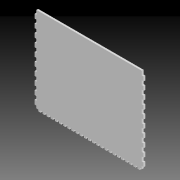
# Autodesk Inventor part: KB33-046-004-016 - Крышка
Saved by Autodesk Inventor 2020 (Build 240168000, 168)
## iProperties
Created: 2021-06-26
Part Number: KB33-046-004-016 - Крышка
Material: Типовые
Document SubType Name: Modeling
Designer: Петров Иван
Mass: 215.32 g
Surface Area: 1127.88 cm^2
Volume: 215.32 cm^3
Density: 1 g/cm^3
Appearance: По умолчанию
Author: Петров Иван
Autodesk Inventor part; units mm, degrees
ref_plane "YZ Plane" through (0, 0, 0) normal (1, 0, 0) x (0, 1, 0)
ref_plane "XZ Plane" through (0, 0, 0) normal (0, 1, 0) x (-1, 0, 0)
ref_plane "XY Plane" through (0, 0, 0) normal (0, 0, 1) x (1, 0, 0)
sketch "Эскиз1" plane through (0, 0, 0) normal (0, 0, 1) x (1, 0, 0)
  line L0 (0, 16.0005) -> (-4, 16.0005) projected
  line L1 (-4, 6.0005) -> (-4, 16.0005) projected
  line L2 (-4, 6.0005) -> (0, 6.0005) projected
  line L3 (0, 16.0005) -> (0, 6.0005) projected
  line L4 (0, 36.0005) -> (-4, 36.0005) projected
  line L5 (-4, 26.0005) -> (-4, 36.0005) projected
  line L6 (-4, 26.0005) -> (0, 26.0005) projected
  line L7 (0, 36.0005) -> (0, 26.0005) projected
  line L8 (0, 56.0005) -> (-4, 56.0005) projected
  line L9 (-4, 46.0005) -> (-4, 56.0005) projected
  line L10 (-4, 46.0005) -> (0, 46.0005) projected
  line L11 (0, 56.0005) -> (0, 46.0005) projected
  line L12 (0, 196.0005) -> (-4, 196.0005) projected
  line L13 (-4, 186.0005) -> (-4, 196.0005) projected
  line L14 (-4, 186.0005) -> (0, 186.0005) projected
  line L15 (0, 196.0005) -> (0, 186.0005) projected
  line L16 (0, 176.0005) -> (-4, 176.0005) projected
  line L17 (-4, 166.0005) -> (-4, 176.0005) projected
  line L18 (-4, 166.0005) -> (0, 166.0005) projected
  line L19 (0, 176.0005) -> (0, 166.0005) projected
  line L20 (0, 156.0005) -> (-4, 156.0005) projected
  line L21 (-4, 146.0005) -> (-4, 156.0005) projected
  line L22 (-4, 146.0005) -> (0, 146.0005) projected
  line L23 (0, 156.0005) -> (0, 146.0005) projected
  line L24 (0, 116.0005) -> (-4, 116.0005) projected
  line L25 (-4, 106.0005) -> (-4, 116.0005) projected
  line L26 (-4, 106.0005) -> (0, 106.0005) projected
  line L27 (0, 116.0005) -> (0, 106.0005) projected
  line L28 (0, 136.0005) -> (-4, 136.0005) projected
  line L29 (-4, 126.0005) -> (-4, 136.0005) projected
  line L30 (-4, 126.0005) -> (0, 126.0005) projected
  line L31 (0, 136.0005) -> (0, 126.0005) projected
  line L32 (0, 96.0005) -> (-4, 96.0005) projected
  line L33 (-4, 86.0005) -> (-4, 96.0005) projected
  line L34 (-4, 86.0005) -> (0, 86.0005) projected
  line L35 (0, 96.0005) -> (0, 86.0005) projected
  line L36 (0, 76.0005) -> (-4, 76.0005) projected
  line L37 (-4, 66.0005) -> (-4, 76.0005) projected
  line L38 (-4, 66.0005) -> (0, 66.0005) projected
  line L39 (0, 76.0005) -> (0, 66.0005) projected
  line L40 (-194, 0) -> (-194, -4) projected
  line L41 (-189, -4) -> (-194, -4) projected
  line L42 (-189, -4) -> (-189, 0) projected
  line L43 (-194, 0) -> (-189, 0) projected
  line L44 (-184, 0) -> (-184, -4) projected
  line L45 (-179, -4) -> (-184, -4) projected
  line L46 (-179, -4) -> (-179, 0) projected
  line L47 (-184, 0) -> (-179, 0) projected
  line L48 (-174, 0) -> (-174, -4) projected
  line L49 (-169, -4) -> (-174, -4) projected
  line L50 (-169, -4) -> (-169, 0) projected
  line L51 (-174, 0) -> (-169, 0) projected
  line L52 (-164, 0) -> (-164, -4) projected
  line L53 (-159, -4) -> (-164, -4) projected
  line L54 (-159, -4) -> (-159, 0) projected
  line L55 (-164, 0) -> (-159, 0) projected
  line L56 (-154, 0) -> (-154, -4) projected
  line L57 (-149, -4) -> (-154, -4) projected
  line L58 (-149, -4) -> (-149, 0) projected
  line L59 (-154, 0) -> (-149, 0) projected
  line L60 (-144, 0) -> (-144, -4) projected
  line L61 (-139, -4) -> (-144, -4) projected
  line L62 (-139, -4) -> (-139, 0) projected
  line L63 (-144, 0) -> (-139, 0) projected
  line L64 (-14, 0) -> (-14, -4) projected
  line L65 (-9, -4) -> (-14, -4) projected
  line L66 (-9, -4) -> (-9, 0) projected
  line L67 (-14, 0) -> (-9, 0) projected
  line L68 (-24, 0) -> (-24, -4) projected
  line L69 (-19, -4) -> (-24, -4) projected
  line L70 (-19, -4) -> (-19, 0) projected
  line L71 (-24, 0) -> (-19, 0) projected
  line L72 (-95.712, 271.7663) -> (-95.712, 277.9752) projected
  line L73 (-34, 0) -> (-34, -4) projected
  line L74 (-29, -4) -> (-34, -4) projected
  line L75 (-29, -4) -> (-29, 0) projected
  line L76 (-34, 0) -> (-29, 0) projected
  line L77 (-44, 0) -> (-44, -4) projected
  line L78 (-39, -4) -> (-44, -4) projected
  line L79 (-39, -4) -> (-39, 0) projected
  line L80 (-44, 0) -> (-39, 0) projected
  line L81 (-54, 0) -> (-54, -4) projected
  line L82 (-49, -4) -> (-54, -4) projected
  line L83 (-49, -4) -> (-49, 0) projected
  line L84 (-54, 0) -> (-49, 0) projected
  line L85 (-64, 0) -> (-64, -4) projected
  line L86 (-59, -4) -> (-64, -4) projected
  line L87 (-59, -4) -> (-59, 0) projected
  line L88 (-64, 0) -> (-59, 0) projected
  line L89 (-74, 0) -> (-74, -4) projected
  line L90 (-69, -4) -> (-74, -4) projected
  line L91 (-69, -4) -> (-69, 0) projected
  line L92 (-74, 0) -> (-69, 0) projected
  line L93 (-84, 0) -> (-84, -4) projected
  line L94 (-79, -4) -> (-84, -4) projected
  line L95 (-79, -4) -> (-79, 0) projected
  line L96 (-84, 0) -> (-79, 0) projected
  line L97 (-94, 0) -> (-94, -4) projected
  line L98 (-89, -4) -> (-94, -4) projected
  line L99 (-89, -4) -> (-89, 0) projected
  line L100 (-94, 0) -> (-89, 0) projected
  line L101 (-104, 0) -> (-104, -4) projected
  line L102 (-99, -4) -> (-104, -4) projected
  line L103 (-99, -4) -> (-99, 0) projected
  line L104 (-104, 0) -> (-99, 0) projected
  line L105 (-114, 0) -> (-114, -4) projected
  line L106 (-109, -4) -> (-114, -4) projected
  line L107 (-109, -4) -> (-109, 0) projected
  line L108 (-114, 0) -> (-109, 0) projected
  line L109 (-134, 0) -> (-134, -4) projected
  line L110 (-129, -4) -> (-134, -4) projected
  line L111 (-129, -4) -> (-129, 0) projected
  line L112 (-134, 0) -> (-129, 0) projected
  line L113 (-124, 0) -> (-124, -4) projected
  line L114 (-119, -4) -> (-124, -4) projected
  line L115 (-119, -4) -> (-119, 0) projected
  line L116 (-124, 0) -> (-119, 0) projected
  line L117 (-259, 16.0005) -> (-263, 16.0005) projected
  line L118 (-263, 6.0005) -> (-263, 16.0005) projected
  line L119 (-263, 6.0005) -> (-259, 6.0005) projected
  line L120 (-259, 16.0005) -> (-259, 6.0005) projected
  line L121 (-259, 36.0005) -> (-263, 36.0005) projected
  line L122 (-263, 26.0005) -> (-263, 36.0005) projected
  line L123 (-263, 26.0005) -> (-259, 26.0005) projected
  line L124 (-259, 36.0005) -> (-259, 26.0005) projected
  line L125 (-259, 56.0005) -> (-263, 56.0005) projected
  line L126 (-263, 46.0005) -> (-263, 56.0005) projected
  line L127 (-263, 46.0005) -> (-259, 46.0005) projected
  line L128 (-259, 56.0005) -> (-259, 46.0005) projected
  line L129 (-259, 76.0005) -> (-263, 76.0005) projected
  line L130 (-263, 66.0005) -> (-263, 76.0005) projected
  line L131 (-263, 66.0005) -> (-259, 66.0005) projected
  line L132 (-259, 76.0005) -> (-259, 66.0005) projected
  line L133 (-259, 96.0005) -> (-263, 96.0005) projected
  line L134 (-263, 86.0005) -> (-263, 96.0005) projected
  line L135 (-263, 86.0005) -> (-259, 86.0005) projected
  line L136 (-259, 96.0005) -> (-259, 86.0005) projected
  line L137 (-259, 116.0005) -> (-263, 116.0005) projected
  line L138 (-263, 106.0005) -> (-263, 116.0005) projected
  line L139 (-263, 106.0005) -> (-259, 106.0005) projected
  line L140 (-259, 116.0005) -> (-259, 106.0005) projected
  line L141 (-259, 136.0005) -> (-263, 136.0005) projected
  line L142 (-263, 126.0005) -> (-263, 136.0005) projected
  line L143 (-263, 126.0005) -> (-259, 126.0005) projected
  line L144 (-259, 136.0005) -> (-259, 126.0005) projected
  line L145 (-259, 156.0005) -> (-259, 146.0005) projected
  line L146 (-259, 156.0005) -> (-263, 156.0005) projected
  line L147 (-263, 146.0005) -> (-263, 156.0005) projected
  line L148 (-263, 146.0005) -> (-259, 146.0005) projected
  line L149 (-259, 156.0005) -> (-259, 146.0005) projected
  line L150 (-259, 176.0005) -> (-263, 176.0005) projected
  line L151 (-263, 166.0005) -> (-263, 176.0005) projected
  line L152 (-263, 166.0005) -> (-259, 166.0005) projected
  line L153 (-259, 176.0005) -> (-259, 166.0005) projected
  line L154 (-259, 196.0005) -> (-259, 186.0005) projected
  line L155 (-259, 196.0005) -> (-263, 196.0005) projected
  line L156 (-263, 186.0005) -> (-263, 196.0005) projected
  line L157 (-263, 186.0005) -> (-259, 186.0005) projected
  line L158 (-259, 196.0005) -> (-259, 186.0005) projected
  line L159 (-4, 196.0005) -> (-4, 206.0005) projected
  line L160 (-4, 196.0005) -> (0, 196.0005) projected
  line L161 (0, 206.0005) -> (0, 196.0005) projected
  line L162 (-4, 206.0005) -> (0, 206.0005) projected
  line L163 (-263, 196.0005) -> (-263, 206.0005) projected
  line L164 (-259, 206.0005) -> (-259, 196.0005) projected
  line L165 (-4, 206.0005) -> (-259, 206.0005)
  line L166 (-259, 206.0005) -> (-259, 0)
  line L167 (-259, 0) -> (-4, 0)
  line L168 (-4, 0) -> (-4, 206.0005)
  line L169 (-204, 0) -> (-204, -4) projected
  line L170 (-199, -4) -> (-204, -4) projected
  line L171 (-199, -4) -> (-199, 0) projected
  line L172 (-204, 0) -> (-199, 0) projected
  line L173 (-214, 0) -> (-214, -4) projected
  line L174 (-209, -4) -> (-214, -4) projected
  line L175 (-209, -4) -> (-209, 0) projected
  line L176 (-214, 0) -> (-209, 0) projected
  line L177 (-224, 0) -> (-224, -4) projected
  line L178 (-219, -4) -> (-224, -4) projected
  line L179 (-219, -4) -> (-219, 0) projected
  line L180 (-224, 0) -> (-219, 0) projected
  line L181 (-234, 0) -> (-234, -4) projected
  line L182 (-229, -4) -> (-234, -4) projected
  line L183 (-229, -4) -> (-229, 0) projected
  line L184 (-234, 0) -> (-229, 0) projected
  line L185 (-244, 0) -> (-244, -4) projected
  line L186 (-239, -4) -> (-244, -4) projected
  line L187 (-239, -4) -> (-239, 0) projected
  line L188 (-244, 0) -> (-239, 0) projected
  line L189 (-253.5, 0) -> (-253.5, -4)
  line L190 (-254, 0) -> (-254, -4) projected
  line L191 (-249, -4) -> (-254, -4) projected
  line L192 (-249, -4) -> (-249, 0) projected
  line L193 (-254, 0) -> (-249, 0) projected
  point P0 (0, 0)
  point P1 (-259, 66.0005)
  point P2 (-259, 56.0005)
  point P3 (-259, 46.0005)
  point P4 (-259, 36.0005)
  point P5 (-259, 26.0005)
  point P6 (-259, 16.0005)
  point P7 (-259, 6.0005)
  point P8 (-199, 206.0005)
  point P9 (-259, 176.0005)
  point P10 (-259, 156.0005)
  point P11 (-259, 146.0005)
  point P12 (-259, 116.0005)
  point P13 (-259, 106.0005)
  point P14 (-259, 96.0005)
  point P15 (-259, 86.0005)
  point P16 (-259, 76.0005)
  constraints: 6 end point, 3 horizontal, 2 vertical, 8 other
extrude "Выдавливание1" add sketch "Эскиз1" along normal blind 4 contours L3 L2 L1 L0 | L1 L168 L167 L67 L71 L76 L80 L84 L88 L92 L96 L100 L104 L108 L116 L112 L63 L59 L55 L51 L47 L43 L166 L120 L124 L128 L132 L136 L140 L144 L145 L153 L154 L164 L165 L159 L13 L17 L21 L29 L25 L33 L37 L9 L5 | L5 L4 L7 L6 | L66 L65 L64 L67 | L9 L8 L11 L10 | L70 L69 L68 L71 | L37 L36 L39 L38 | L75 L74 L73 L76 | L33 L32 L35 L34 | L79 L78 L77 L80 | L25 L24 L27 L26 | L83 L82 L81 L84 | L29 L28 L31 L30 | L87 L86 L85 L88 | L21 L20 L23 L22 | L91 L90 L89 L92 | L17 L16 L19 L18 | L95 L94 L93 L96 | L13 L12 L15 L14 | L99 L98 L97 L100 | L103 L102 L101 L104 | L154 L157 L156 L155 | L107 L106 L105 L108 | L153 L152 L151 L150 | L115 L114 L113 L116 | L145 L148 L147 L146 | L111 L110 L109 L112 | L144 L143 L142 L141 | L62 L61 L60 L63 | L140 L139 L138 L137 | L58 L57 L56 L59 | L136 L135 L134 L133 | L54 L53 L52 L55 | L132 L131 L130 L129 | L50 L49 L48 L51 | L128 L127 L126 L125 | L46 L45 L44 L47 | L124 L123 L122 L121 | L42 L41 L40 L43 | L120 L119 L118 L117 | L171 L170 L169 L167 | L167 L189 L191 L190 | L175 L174 L173 L167 | L167 L192 L191 L189 | L179 L178 L177 L167 | L167 L187 L186 L185 | L183 L182 L181 L167
